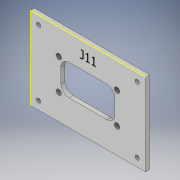
# Autodesk Inventor part: LFEV2017_TSI_007
Saved by Autodesk Inventor 2017 (Build 210142000, 142)
## iProperties
Created: 2017-03-22
Part Number: LFEV2017_TSI_007
Material: Generic
Document SubType Name: Modeling
Designer: hoeflinc
Density: 1 g/cm^3
Appearance: Default
Author: hoeflinc
Autodesk Inventor part; units mm, degrees
ref_plane "YZ Plane" through (0, 0, 0) normal (1, 0, 0) x (0, 1, 0)
ref_plane "XZ Plane" through (0, 0, 0) normal (0, 1, 0) x (-1, 0, 0)
ref_plane "XY Plane" through (0, 0, 0) normal (0, 0, 1) x (1, 0, 0)
sketch "Sketch1" plane through (0, 0, 0) normal (0, 0, 1) x (1, 0, 0)
  line L0 (0, 0) -> (88.9, 0)
  line L1 (88.9, 0) -> (88.9, 63.5)
  line L2 (88.9, 63.5) -> (0, 63.5)
  line L3 (0, 63.5) -> (0, 0)
  dimension "d0" = 88.9
  dimension "d1" = 63.5
  constraints: 8 end point, 2 parallel, 1 horizontal, 1 perpendicular
  measures "d0" distance of L1.end L2.end
  measures "d1" distance of L2.end L0.start
extrude "Extrusion1" add sketch "Sketch1" along normal blind 3.175
sketch "Sketch2" plane through (0, 0, 3.175) normal (0, 0, 1) x (1, 0, 0)
  line L0 (16.891, 13.97) -> (72.009, 13.97)
  line L1 (72.009, 13.97) -> (72.009, 49.53)
  line L2 (72.009, 49.53) -> (16.891, 49.53)
  line L3 (16.891, 49.53) -> (16.891, 13.97)
  circle A0 centre (21.971, 43.688) radius 2.0828
  circle A1 centre (66.929, 43.688) radius 2.0828
  circle A2 centre (66.929, 19.812) radius 2.0828
  circle A3 centre (21.971, 19.812) radius 2.0828
  line L4 (29.8704, 19.9898) -> (59.0042, 19.9898)
  line L5 (65.3542, 26.3398) -> (65.3542, 37.5158)
  line L6 (59.0042, 43.8658) -> (29.8704, 43.8658)
  line L7 (23.5204, 37.5158) -> (23.5204, 26.3398)
  arc A4 (29.8704, 43.8658) -> (23.5204, 37.5158) centre (29.8704, 37.5158) ccw
  arc A5 (23.5204, 26.3398) -> (29.8704, 19.9898) centre (29.8704, 26.3398) ccw
  arc A6 (59.0042, 19.9898) -> (65.3542, 26.3398) centre (59.0042, 26.3398) ccw
  arc A7 (65.3542, 37.5158) -> (59.0042, 43.8658) centre (59.0042, 37.5158) ccw
  line L8 (0, 63.5) -> (0, 0) projected
  line L9 (88.9, 0) -> (88.9, 63.5) projected
  line L10 (0, 0) -> (88.9, 0) projected
  line L11 (88.9, 63.5) -> (0, 63.5) projected
  point P0 (23.5204, 19.9898)
  point P1 (65.3542, 43.8658)
  point P2 (65.3542, 19.9898)
  dimension "d4" = 55.118
  dimension "d5" = 35.56
  dimension "d6" = 4.1656
  dimension "d7" = 5.08
  dimension "d8" = 5.842
  dimension "d9" = 5.842
  dimension "d10" = 5.842
  dimension "d11" = 5.842
  dimension "d12" = 5.08
  dimension "d13" = 5.08
  dimension "d14" = 5.08
  dimension "d15" = 23.876
  dimension "d16" = 41.8338
  dimension "d17" = 1.5748
  dimension "d18" = 0.1778
  dimension "d19" = 6.35
  dimension "d20" = 88.9
  dimension "d21" = 63.5
  dimension "d22" = 13.97
  dimension "d23" = 16.891
  constraints: 16 end point, 8 centre point, 8 point on circle, 8 tangent, 6 equal radius, 6 point on line, 4 parallel, 2 horizontal, 2 perpendicular
  measures "d4" distance of L1.end L3.start
  measures "d5" distance of L3.start L0.start
  measures "d6" diameter of A1
  measures "d7" distance from line of L1 A1.centre
  measures "d8" distance from line of L2 A1.centre
  measures "d9" distance from line of L2 A0.centre
  measures "d10" distance from line of L0 A3.centre
  measures "d11" distance from line of A2.centre L0
  measures "d12" distance from line of L1 A2.centre
  measures "d13" distance from line of L3 A3.centre
  measures "d14" distance from line of L3 A0.centre
  measures "d15" distance of point (65.354, 19.99) point (65.354, 43.866)
  measures "d16" distance of point (23.52, 19.99) point (65.354, 19.99)
  measures "d17" distance from line of A1.centre L5
  measures "d18" distance from line of A2.centre L4
  measures "d19" radius of A4
  measures "d20" distance between parallel lines of L8 L9
  measures "d21" distance between parallel lines of L10 L11
  measures "d22" distance between parallel lines of L11 L2
  measures "d23" distance between parallel lines of L9 L1
extrude "Extrusion2" cut sketch "Sketch2" against normal through all contours A0 | A1 | A2 | A3 | A5 L7 A4 L6 A7 L5 A6 L4
sketch "Sketch4" plane through (0, 0, 3.175) normal (0, 0, 1) x (1, 0, 0)
  line L0 (38.1, 57.15) -> (51.2683, 57.15) construction
  line L1 (51.2683, 57.15) -> (51.2683, 45.6081) construction
  line L2 (51.2683, 45.6081) -> (38.1, 45.6081) construction
  line L3 (38.1, 45.6081) -> (38.1, 57.15) construction
  line L4 (0, 63.5) -> (0, 0) projected
  line L5 (88.9, 63.5) -> (0, 63.5) projected
  constraints: 2 other
sketch "Sketch5" plane through (0, 0, 0) normal (0, 0, -1) x (-1, 0, 0)
  line L0 (-61.8811, 60.2648) -> (-25.8263, 60.2648) construction
  line L1 (-25.8263, 60.2648) -> (-25.8263, 56.54) construction
  line L2 (-25.8263, 56.54) -> (-61.8811, 56.54) construction
  line L3 (-61.8811, 56.54) -> (-61.8811, 60.2648) construction
  point P0 (0, 0)
  constraints: 2 other
sketch "Sketch6" plane through (0, 0, 3.175) normal (0, 0, 1) x (1, 0, 0)
  line L0 (0, 63.5) -> (0, 0) projected
  circle A0 centre (66.929, 43.688) radius 2.0828 projected
  circle A1 centre (21.971, 19.812) radius 2.0828 projected
  circle A2 centre (21.971, 43.688) radius 2.0828 projected
  circle A3 centre (66.929, 19.812) radius 2.0828 projected
  arc A4 (59.0042, 19.9898) -> (65.3542, 26.3398) centre (59.0042, 26.3398) ccw projected
  line L1 (59.0042, 19.9898) -> (29.8704, 19.9898) projected
  arc A5 (23.5204, 26.3398) -> (29.8704, 19.9898) centre (29.8704, 26.3398) ccw projected
  line L2 (23.5204, 26.3398) -> (23.5204, 37.5158) projected
  arc A6 (29.8704, 43.8658) -> (23.5204, 37.5158) centre (29.8704, 37.5158) ccw projected
  line L3 (29.8704, 43.8658) -> (59.0042, 43.8658) projected
  arc A7 (65.3542, 37.5158) -> (59.0042, 43.8658) centre (59.0042, 37.5158) ccw projected
  line L4 (65.3542, 37.5158) -> (65.3542, 26.3398) projected
  line L5 (0, 0) -> (88.9, 0) projected
  line L6 (88.9, 0) -> (88.9, 63.5) projected
  line L7 (88.9, 63.5) -> (0, 63.5) projected
  line L8 (0, 63.5) -> (0, 0) projected
  point P0 (6.35, 57.15)
  point P1 (82.55, 57.15)
  point P2 (82.55, 6.35)
  point P3 (6.35, 6.35)
  dimension "d57" = 6.35
  dimension "d58" = 6.35
  dimension "d59" = 6.35
  dimension "d60" = 6.35
  dimension "d61" = 6.35
  dimension "d62" = 6.35
  dimension "d63" = 6.35
  dimension "d64" = 6.35
  measures "d57" distance from line of L0 point (6.35, 57.15)
  measures "d58" distance from line of L7 point (6.35, 57.15)
  measures "d59" distance from line of L7 point (82.55, 57.15)
  measures "d60" distance from line of point (82.55, 57.15) L6
  measures "d61" distance from line of L6 point (82.55, 6.35)
  measures "d62" distance from line of point (82.55, 6.35) L5
  measures "d63" distance from line of point (6.35, 6.35) L5
  measures "d64" distance from line of L0 point (6.35, 6.35)
hole "Hole1" at (6.35, 57.15, 3.175) at (6.35, 6.35, 3.175) at (82.55, 6.35, 3.175) at (82.55, 57.15, 3.175) direction (0, 0, -1) diameter 3.302 end through all
thread "Thread9" size "8-32 UNC" class "2B" standard "ANSI Unified Screw Threads" full length
thread "Thread10" size "8-32 UNC" class "2B" standard "ANSI Unified Screw Threads" full length
thread "Thread11" size "8-32 UNC" class "2B" standard "ANSI Unified Screw Threads" full length
thread "Thread12" size "8-32 UNC" class "2B" standard "ANSI Unified Screw Threads" full length
equation "\"d9\" = d8"
equation "\"d10\" = d9"
equation "\"d11\" = d8"
equation "\"d12\" = d7"
equation "\"d13\" = d7"
equation "\"d14\" = d7"
equation "\"d22\" = -0.5 * d5 + 0.5 * d21"
equation "\"d23\" = -0.5 * d4 + 0.5 * d20"
equation "\"d58\" = d57"
equation "\"d59\" = d58"
equation "\"d60\" = d59"
equation "\"d61\" = d59"
equation "\"d62\" = d61"
equation "\"d63\" = d58"
equation "\"d64\" = d63"
body "Solid1"
